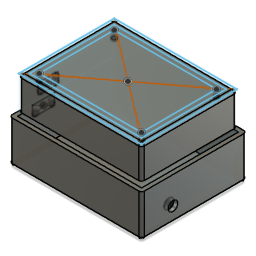
fsk-traffic-controller (Autodesk Fusion 360 design; units mm, degrees)
Autodesk Fusion 360 part; units mm, degrees
note: some values were not read from the file. Set by a fixed rule: which sketch regions a step uses.
sketch "스케치1" plane through (0, 0, 0) normal (0, 1, 0) x (1, 0, 0)
  line L0 (105.4333, -69.5) -> (8.4333, -69.5)
  line L1 (8.4333, -69.5) -> (8.4333, 7.5)
  line L2 (8.4333, 7.5) -> (105.4333, 7.5)
  line L3 (105.4333, 7.5) -> (105.4333, -69.5)
  line L4 (105.4333, -69.5) -> (8.4333, 7.5) construction
  line L5 (8.4333, -69.5) -> (105.4333, 7.5) construction
  line L6 (102.4333, -66.5) -> (11.4333, -66.5)
  line L7 (11.4333, -66.5) -> (11.4333, 4.5)
  line L8 (11.4333, 4.5) -> (102.4333, 4.5)
  line L9 (102.4333, 4.5) -> (102.4333, -66.5)
  line L10 (102.4333, -66.5) -> (11.4333, 4.5) construction
  line L11 (11.4333, -66.5) -> (102.4333, 4.5) construction
  line L12 (11.4333, 4.5) -> (15.4333, 4.5)
  line L13 (15.4333, 4.5) -> (15.4333, 0.5)
  line L14 (15.4333, 0.5) -> (11.4333, 0.5)
  line L15 (11.4333, 0.5) -> (11.4333, 4.5)
  line L16 (102.4333, 4.5) -> (98.4333, 4.5)
  line L17 (98.4333, 4.5) -> (98.4333, 0.5)
  line L18 (98.4333, 0.5) -> (102.4333, 0.5)
  line L19 (102.4333, 0.5) -> (102.4333, 4.5)
  line L20 (11.4333, -66.5) -> (15.4333, -66.5)
  line L21 (15.4333, -66.5) -> (15.4333, -62.5)
  line L22 (15.4333, -62.5) -> (11.4333, -62.5)
  line L23 (11.4333, -62.5) -> (11.4333, -66.5)
  line L24 (102.4333, -66.5) -> (98.4333, -66.5)
  line L25 (98.4333, -66.5) -> (98.4333, -62.5)
  line L26 (98.4333, -62.5) -> (102.4333, -62.5)
  line L27 (102.4333, -62.5) -> (102.4333, -66.5)
  point P0 (56.9333, -31)
  point P1 (56.9333, -31)
  point P2 (56.9333, -31)
  dimension "d9" = 97
  dimension "d10" = 77
  dimension "d11" = 91
  dimension "d12" = 71
  dimension "d51" = 4
  dimension "d52" = 4
  dimension "d53" = 4
  dimension "d54" = 4
  dimension "d55" = 4
  dimension "d56" = 4
  dimension "d57" = 4
  dimension "d60" = 4
  constraint horizontal L0
  constraint perpendicular L0 L1
  constraint parallel L0 L2
  constraint parallel L1 L3
  constraint coincident L4 P2
  constraint coincident L5 P2
  constraint horizontal L6
  constraint perpendicular L6 L7
  constraint parallel L6 L8
  constraint parallel L7 L9
  constraint coincident L10 P2
  constraint coincident L11 P2
  constraint coincident P2 P1
  constraint horizontal L12
  constraint vertical L13
  constraint horizontal L14
  constraint vertical L15
  constraint horizontal L16
  constraint vertical L17
  constraint horizontal L18
  constraint vertical L19
  constraint horizontal L20
  constraint vertical L21
  constraint horizontal L22
  constraint vertical L23
  constraint horizontal L24
  constraint vertical L25
  constraint horizontal L26
  constraint vertical L27
  measures "d9" distance of L1.end L2.end
  measures "d10" distance of L0.end L1.end
  measures "d11" distance of L7.end L8.end
  measures "d12" distance of L6.end L7.end
  measures "d51" distance of L7.end L12.end
  measures "d52" distance of L7.end L14.end
  measures "d53" distance of L8.end L16.end
  measures "d54" distance of L8.end L18.end
  measures "d55" distance of L6.end L20.end
  measures "d56" distance of L6.start L24.end
  measures "d57" distance of L6.start L26.end
  measures "d60" distance of L20 L22
extrude "돌출6" add sketch "스케치1" along normal blind 4 contours L0 L1 L2 L3 | L6 L9 L24 L25 L26 L27 | L6 L7 L8 L9 L13 L14 L17 L18 L21 L22 L25 L26 | L6 L7 L20 L21 L22 L23 | L8 L9 L16 L17 L18 L19 | L7 L8 L12 L13 L14 L15 makes body 1
extrude "돌출7" add sketch "스케치1" along normal blind 34 bodies 1
fillet "필렛3" radius 2 4 edges at (105.4333, 17, -7.5) (105.4333, 17, 69.5) (8.4333, 17, -7.5) (8.4333, 17, 69.5) on bodies 1
extrude "돌출8" add sketch "스케치1" along normal blind 20 contours L6 L9 L24 L25 L26 L27 | L6 L7 L20 L21 L22 L23 | L8 L9 L16 L17 L18 L19 | L7 L8 L12 L13 L14 L15 bodies 1
sketch "스케치4" plane through (102.4333, 0, 0) normal (-1, 0, 0) x (0, 0, 1)
  line L0 (-4.5, 20) -> (-0.5, 20)
  line L1 (-0.5, 20) -> (-0.5, 4)
  line L2 (-0.5, 4) -> (62.5, 4)
  line L3 (62.5, 4) -> (62.5, 20)
  line L4 (62.5, 20) -> (66.5, 20)
  line L5 (66.5, 20) -> (66.5, 34)
  line L6 (66.5, 34) -> (-4.5, 34)
  line L7 (-4.5, 34) -> (-4.5, 20)
  circle A0 centre (46.5, 12) radius 3.5
  dimension "d61" = 7
  dimension "d62" = 20
  dimension "d63" = 8
  measures "d61" diameter of A0
  measures "d62" distance of L5 A0.centre
  measures "d63" distance of L2 A0.centre
extrude "돌출9" cut sketch "스케치4" against normal blind 10 contours A0 bodies 1
fillet "필렛4" radius 2 8 edges at (104.8475, 0, -6.9142) (105.4333, 0, 31) (104.8475, 0, 68.9142) (56.9333, 0, 69.5) (9.0191, 0, 68.9142) (8.4333, 0, 31) (9.0191, 0, -6.9142) (56.9333, 0, -7.5) on bodies 1
extrude "돌출10" cut 1 faces at (41.7666, 34, -6.5) along direction (0, -1, 0) blind 2 on bodies 1 bodies 1
extrude "돌출11" cut sketch "스케치1" along normal blind 2 bodies 1
extrude "돌출12" add 1 faces at (41.7666, 2, -6.5) along direction (0, -1, 0) blind 1 on bodies 1 bodies 1
sketch "스케치5" plane through (0, 0, 0) normal (0, -1, 0) x (1, 0, 0)
  line L0 (11.4333, -4.5) -> (102.4333, -4.5)
  line L1 (102.4333, -4.5) -> (102.4333, 66.5)
  line L2 (102.4333, 66.5) -> (11.4333, 66.5)
  line L3 (11.4333, 66.5) -> (11.4333, -4.5)
extrude "돌출13" cut sketch "스케치5" against normal blind 1 bodies 1
fillet "필렛5" radius 2 8 edges at (8.4333, 1, 31) (9.0191, 1, -6.9142) (56.9333, 1, -7.5) (104.8475, 1, -6.9142) (105.4333, 1, 31) (104.8475, 1, 68.9142) (56.9333, 1, 69.5) (9.0191, 1, 68.9142) on bodies 1
sketch "스케치6" plane through (8.4333, 0, 0) normal (-1, 0, 0) x (0, 0, 1)
  line L0 (-5.5, 3) -> (67.5, 3)
  line L1 (67.5, 3) -> (67.5, 32)
  line L2 (67.5, 32) -> (-5.5, 32)
  line L3 (-5.5, 32) -> (-5.5, 3)
  line L4 (36.5, 30.5) -> (52.5, 30.5)
  line L5 (52.5, 30.5) -> (52.5, 24.5)
  line L6 (50.5, 22.5) -> (38.5, 22.5)
  line L7 (36.5, 24.5) -> (36.5, 30.5)
  line L8 (36.5, 30.5) -> (52.5, 22.5) construction
  line L9 (52.5, 30.5) -> (36.5, 22.5) construction
  arc A0 (50.5, 22.5) -> (52.5, 24.5) centre (50.5, 24.5) ccw
  arc A1 (36.5, 24.5) -> (38.5, 22.5) centre (38.5, 24.5) ccw
  point P0 (44.5, 26.5)
  dimension "d78" = 16
  dimension "d79" = 23
  dimension "d80" = 5.5
  dimension "d81" = 8
  dimension "d90" = 2
  dimension "d91" = 2
  constraint horizontal L4
  constraint perpendicular L4 L5
  constraint parallel L4 L6
  constraint parallel L5 L7
  constraint coincident L8 P0
  constraint coincident L9 P0
  constraint coincident L8.end L5
  constraint coincident L8.end L6
  constraint tangent L5 A0
  constraint tangent L6 A0
  constraint coincident L9.end L6
  constraint coincident L9.end L7
  constraint tangent L6 A1
  constraint tangent L7 A1
  measures "d78" distance of L8.end L9.end
  measures "d79" distance of L1 P0
  measures "d80" distance of L2 P0
  measures "d81" distance of L4 L6
  measures "d90" radius of A0
  measures "d91" radius of A1
extrude "돌출14" cut sketch "스케치6" against normal blind 10 contours L4 L5 L6 L7 A0 A1 bodies 1
extrude "돌출15" cut 1 faces at (9.4333, 30.5, 47.1667) along direction (0, 1, 0) blind 10 on bodies 1 bodies 1
fillet "필렛6" radius 1 2 edges at (9.9333, 32, 52.5) (9.9333, 32, 36.5) on bodies 1
fillet "필렛7" [no effect]
sketch "스케치1 (2)" plane through (0, 0, 0) normal (0, 1, 0) x (1, 0, 0) in component "fsk-traffic-controller-base v3"
  line L0 (94, -66) -> (4, -66)
  line L1 (4, -66) -> (4, 4)
  line L2 (4, 4) -> (94, 4)
  line L3 (94, 4) -> (94, -66)
  line L4 (94, -66) -> (4, 4) construction
  line L5 (4, -66) -> (94, 4) construction
  line L6 (90, -62) -> (8, -62)
  line L7 (8, -62) -> (8, 0)
  line L8 (8, 0) -> (90, 0)
  line L9 (90, 0) -> (90, -62)
  line L10 (90, -62) -> (8, 0) construction
  line L11 (8, -62) -> (90, 0) construction
  line L12 (86.5, -58.5) -> (11.5, -58.5)
  line L13 (11.5, -58.5) -> (11.5, -3.5)
  line L14 (11.5, -3.5) -> (86.5, -3.5)
  line L15 (86.5, -3.5) -> (86.5, -58.5)
  line L16 (86.5, -58.5) -> (11.5, -3.5) construction
  line L17 (11.5, -58.5) -> (86.5, -3.5) construction
  circle A0 centre (11.5, -3.5) radius 2.2
  circle A1 centre (86.5, -3.5) radius 2.2
  circle A2 centre (11.5, -58.5) radius 2.2
  circle A3 centre (86.5, -58.5) radius 2.2
  point P0 (49, -31)
  point P1 (49, -31)
  point P2 (49, -31)
  dimension "d9_1" = 90
  dimension "d10_1" = 70
  dimension "d11_1" = 82
  dimension "d12_1" = 62
  dimension "d13" = 75
  dimension "d14" = 55
  dimension "d15" = 4.4
  dimension "d16" = 4.4
  dimension "d17" = 4.4
  dimension "d18" = 4.4
  constraint horizontal L0
  constraint perpendicular L0 L1
  constraint parallel L0 L2
  constraint parallel L1 L3
  constraint coincident L4 P2
  constraint coincident L5 P2
  constraint horizontal L6
  constraint perpendicular L6 L7
  constraint parallel L6 L8
  constraint parallel L7 L9
  constraint coincident L10 P2
  constraint coincident L11 P2
  constraint coincident P2 P1
  constraint horizontal L12
  constraint perpendicular L12 L13
  constraint parallel L12 L14
  constraint parallel L13 L15
  constraint coincident L16 P2
  constraint coincident L17 P2
  constraint coincident L13.end L14.start
  constraint coincident L14.end L15.start
  constraint coincident L12.end L13.start
  constraint coincident L12.start L15.end
  measures "d9_1" distance of L1.end L2.end
  measures "d10_1" distance of L0.end L1.end
  measures "d11_1" distance of L7.end L8.end
  measures "d12_1" distance of L6.end L7.end
  measures "d13" distance of L13.end L14.end
  measures "d14" distance of L12.end L13.end
  measures "d15" diameter of A0
  measures "d16" diameter of A1
  measures "d17" diameter of A2
  measures "d18" diameter of A3
extrude "돌출1" add sketch "스케치1 (2)" along normal blind 3.6 separate body contours L0 L1 L2 L3 | L6 L7 L8 L9 | L12 L13 L14 L15 A0 A1 A2 A3 makes body 2 in component "fsk-traffic-controller-base v3"
extrude "돌출2" add sketch "스케치1 (2)" along normal blind 24 contours L0 L1 L2 L3 bodies 2 in component "fsk-traffic-controller-base v3"
extrude "돌출3" add 1 faces at (37.1059, 3.6, 39.7536) along direction (0, 1, 0) blind 1.4 on bodies 2 bodies 2 in component "fsk-traffic-controller-base v3"
sketch "스케치2" plane through (0, 5, 0) normal (0, 1, 0) x (-1, 0, 0) in component "fsk-traffic-controller-base v3"
  line L0 (-8, 0) -> (-8, 62)
  line L1 (-8, 62) -> (-90, 62)
  line L2 (-90, 62) -> (-90, 0)
  line L3 (-90, 0) -> (-8, 0)
  circle A0 centre (-11.5, 3.5) radius 2.2
  circle A1 centre (-86.5, 3.5) radius 2.2
  circle A2 centre (-11.5, 58.5) radius 2.2
  circle A3 centre (-86.5, 58.5) radius 2.2
  circle A4 centre (-11.5, 3.5) radius 1.5
  circle A5 centre (-86.5, 3.5) radius 1.5
  circle A6 centre (-86.5, 58.5) radius 1.5
  circle A7 centre (-11.5, 58.5) radius 1.5
  dimension "d25" = 3
  dimension "d26" = 3
  dimension "d27" = 3
  dimension "d28" = 3
  constraint concentric A0 A4
  constraint concentric A1 A5
  constraint concentric A3 A6
  constraint concentric A2 A7
  measures "d25" diameter of A4
  measures "d26" diameter of A5
  measures "d27" diameter of A6
  measures "d28" diameter of A7
extrude "돌출4" add sketch "스케치2" against normal blind 2.5 contours A0 | A1 | A2 | A3 bodies 2 in component "fsk-traffic-controller-base v3"
sketch "스케치3" plane through (94, 0, 0) normal (1, 0, 0) x (0, 0, -1) in component "fsk-traffic-controller-base v3"
  line L0 (-66, 0) -> (4, 0)
  line L1 (4, 0) -> (4, 24)
  line L2 (4, 24) -> (-66, 24)
  line L3 (-66, 24) -> (-66, 0)
  line L4 (-39, 13) -> (-50, 13)
  line L5 (-52, 15) -> (-52, 19)
  line L6 (-50, 21) -> (-39, 21)
  line L7 (-37, 19) -> (-37, 15)
  line L8 (-37, 13) -> (-52, 21) construction
  line L9 (-52, 13) -> (-37, 21) construction
  arc A0 (-37, 19) -> (-39, 21) centre (-39, 19) ccw
  arc A1 (-39, 13) -> (-37, 15) centre (-39, 15) ccw
  arc A2 (-50, 21) -> (-52, 19) centre (-50, 19) ccw
  arc A3 (-52, 15) -> (-50, 13) centre (-50, 15) ccw
  point P0 (-44.5, 17)
  dimension "d31" = 15
  dimension "d32" = 8
  dimension "d33" = 21.5
  dimension "d34" = 7
  dimension "d35" = 2
  dimension "d36" = 2
  dimension "d37" = 2
  dimension "d38" = 2
  constraint horizontal L4
  constraint perpendicular L4 L5
  constraint parallel L4 L6
  constraint parallel L5 L7
  constraint coincident L8 P0
  constraint coincident L9 P0
  constraint coincident L9.end L7
  constraint coincident L9.end L6
  constraint tangent L7 A0
  constraint tangent L6 A0
  constraint coincident L8.start L7
  constraint coincident L8.start L4
  constraint tangent L7 A1
  constraint tangent L4 A1
  constraint coincident L8.end L6
  constraint coincident L8.end L5
  constraint tangent L6 A2
  constraint tangent L5 A2
  constraint coincident L9.start L5
  constraint coincident L9.start L4
  constraint tangent L5 A3
  constraint tangent L4 A3
  measures "d31" distance of L8.end L9.end
  measures "d32" distance of L9.start L8.end
  measures "d33" distance of L3 P0
  measures "d34" distance of L2 P0
  measures "d35" radius of A0
  measures "d36" radius of A1
  measures "d37" radius of A2
  measures "d38" radius of A3
extrude "돌출5" cut sketch "스케치3" against normal blind 5 contours L4 L5 L6 L7 A0 A1 A2 A3 bodies 2 in component "fsk-traffic-controller-base v3"
fillet "필렛1" radius 2 4 edges at (94, 12, 66) (94, 12, -4) (4, 12, -4) (4, 12, 66) on bodies 2 in component "fsk-traffic-controller-base v3"
fillet "필렛2" radius 2 8 edges at (4.5858, 0, -3.4142) (49, 0, -4) (93.4142, 0, -3.4142) (94, 0, 31) (93.4142, 0, 65.4142) (49, 0, 66) (4.5858, 0, 65.4142) (4, 0, 31) on bodies 2 in component "fsk-traffic-controller-base v3"
move_body "이동1" bodies 2 to x (1, 0, 0) y (0, 1, 0) z (0, 0, 1) at (0, 13, 0) in component "fsk-traffic-controller-base v3"
delete_face "면 삭제1" 1 faces at (10.4333, 31.8888, 53.0418) on bodies 1
delete_face "면 삭제2" 1 faces at (10.4333, 31.5801, 36.3146) on bodies 1
fillet "필렛8" radius 2 1 edges at (9.9333, 32, 52.5) on bodies 1
fillet "필렛9" radius 2 1 edges at (9.9333, 32, 36.5) on bodies 1
move_body "이동2" bodies 2 to x (1, 0, 0) y (0, 1, 0) z (0, 0, 1) at (0, -13, 0) in component "fsk-traffic-controller-base v3"
component "fsk-traffic-controller-base v3" placed x (-1, 0, 0) y (0, -1, 0) z (0, 0, 1) at (105.8421, 44.1181, 0)
